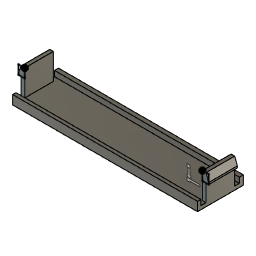
clone-bay-cover-3.5 (Autodesk Fusion 360 design; units mm, degrees)
Autodesk Fusion 360 part; units mm, degrees
sketch "Base" plane through (0, 0, 0) normal (0, 0, 1) x (1, 0, 0)
  line L0 (2, 2) -> (105.25, 2)
  line L1 (105.25, 2) -> (105.25, 27.6)
  line L2 (105.25, 27.6) -> (2, 27.6)
  line L3 (2, 27.6) -> (2, 2)
  dimension "d1" = 25.6
  dimension "d2" = 103.25
  constraint horizontal L0
  constraint vertical L1
  constraint horizontal L2
  constraint vertical L3
  measures "d1" distance of L0.start L2.end
  measures "d2" distance of L0.start L0.end
  measures "d15" distance of L0.start
extrude "Extrude1" add sketch "Base" along normal blind 2
sketch "Rail" plane through (0, 0, 2) normal (0, 0, 1) x (-1, 0, 0)
  line L0 (-2, -27.6) -> (-2, -2)
  line L1 (-2, -2) -> (-105.25, -2)
  line L2 (-105.25, -2) -> (-105.25, -27.6)
  line L3 (-105.25, -27.6) -> (-2, -27.6)
  line L4 (-2, -27.6) -> (-105.25, -27.6)
  line L5 (-105.25, -27.6) -> (-105.25, -25.35)
  line L6 (-105.25, -25.35) -> (-2, -25.35)
  line L7 (-2, -25.35) -> (-2, -27.6)
  line L8 (-2, -2) -> (-105.25, -2)
  line L9 (-105.25, -2) -> (-105.25, -3.88)
  line L10 (-105.25, -3.88) -> (-2, -3.88)
  line L11 (-2, -3.88) -> (-2, -2)
  dimension "d5" = 2.25
  dimension "d6" = 1.88
  constraint horizontal L4
  constraint vertical L5
  constraint horizontal L6
  constraint vertical L7
  constraint coincident L2 L5.end
  constraint coincident L0.start L3.end
  constraint horizontal L8
  constraint vertical L9
  constraint horizontal L10
  constraint vertical L11
  constraint coincident L2 L9.end
  constraint coincident L0.end L1.start
  measures "d5" distance of L4 L6
  measures "d6" distance of L8 L10
extrude "Extrude2" add sketch "Rail" along normal blind 3 contours L0 L2 L3 L4 L5 L6 L7 | L0 L1 L2 L8 L9 L10 L11
sketch "Hook (1.5mm -> 2mm)" plane through (0, 0, 2) normal (0, 0, 1) x (-1, 0, 0)
  line L0 (-2, -3.88) -> (-105.25, -3.88)
  line L1 (-105.25, -3.88) -> (-105.25, -25.35)
  line L2 (-105.25, -25.35) -> (-2, -25.35)
  line L3 (-2, -25.35) -> (-2, -3.88)
  line L4 (-2, -22.75) -> (-4, -22.75)
  line L5 (-4, -22.75) -> (-4, -6.75)
  line L6 (-4, -6.75) -> (-2, -6.75)
  line L7 (-2, -6.75) -> (-2, -22.75)
  line L8 (-105.25, -22.75) -> (-103.25, -22.75)
  line L9 (-103.25, -22.75) -> (-103.25, -6.75)
  line L10 (-103.25, -6.75) -> (-105.25, -6.75)
  line L11 (-105.25, -6.75) -> (-105.25, -22.75)
  dimension "d9" = 2.6
  dimension "d10" = 16
  dimension "d11" = 3.07
  dimension "d12" = 2
  dimension "d13" = 2
  dimension "d14" = 16
  dimension "d15" = 2.6
  dimension "d16" = 2.87
  constraint horizontal L4
  constraint vertical L5
  constraint horizontal L6
  constraint vertical L7
  constraint coincident L3 L4.start
  constraint horizontal L8
  constraint vertical L9
  constraint horizontal L10
  constraint vertical L11
  constraint coincident L1 L8.start
  measures "d9" distance of L2 L4
  measures "d10" distance of L4 L6
  measures "d12" distance of L5 L7
  measures "d13" distance of L8.start L8.end
  measures "d14" distance of L8.start L10.end
  measures "d15" distance of L2 L8.start
  measures "d16" distance of L0 L9.end
extrude "Extrude3" add sketch "Hook (1.5mm -> 2mm)" along normal blind 14.5 contours L3 L4 L5 L6 L7 | L1 L8 L9 L10 L11
sketch "Hook Left" plane through (0, 6.75, 0) normal (0, -1, 0) x (1, 0, 0)
  line L0 (2, 2) -> (4, 2)
  line L1 (4, 2) -> (4, 16.5)
  line L2 (4, 16.5) -> (2, 16.5)
  line L3 (2, 16.5) -> (2, 2)
  line L4 (4, 16.5) -> (0.5, 16.5)
  line L5 (0.5, 16.5) -> (0.5, 11.5)
  line L6 (0.5, 11.5) -> (4, 11.5)
  line L7 (4, 11.5) -> (4, 16.5)
  dimension "d19" = 3.5
  dimension "d20" = 5
  constraint horizontal L4
  constraint vertical L5
  constraint horizontal L6
  constraint vertical L7
  constraint coincident L1.end L2.start
  measures "d19" distance of L1.end L4.end
  measures "d20" distance of L1.end L6.end
sketch "Hook Right" plane through (0, 6.75, 0) normal (0, -1, 0) x (1, 0, 0)
  line L0 (103.25, 2) -> (105.25, 2)
  line L1 (105.25, 2) -> (105.25, 16.5)
  line L2 (105.25, 16.5) -> (103.25, 16.5)
  line L3 (103.25, 16.5) -> (103.25, 2)
  line L4 (103.25, 16.5) -> (106.75, 16.5)
  line L5 (106.75, 16.5) -> (106.75, 11.5)
  line L6 (106.75, 11.5) -> (103.25, 11.5)
  line L7 (103.25, 11.5) -> (103.25, 16.5)
  dimension "d21" = 5
  dimension "d22" = 3.5
  constraint horizontal L4
  constraint vertical L5
  constraint horizontal L6
  constraint vertical L7
  constraint coincident L2.end L3.start
  measures "d21" distance of L2.end L6.end
  measures "d22" distance of L2.end L4.end
extrude "Extrude5" add sketch "Hook Left" sketch "Hook Right" against normal blind 16 contours L3 L4 L5 L6 of sketch 2 contours L1 L4 L5 L6
chamfer "Chamfer1" distance 4 distance2 1.5 1 edges at (0.5, 14.75, 16.5) measured on face at (0.5, 12.0833, 14.8333)
chamfer "Chamfer2" distance 1.5 distance2 4 1 edges at (106.75, 14.75, 16.5) measured on face at (104.4167, 12.0833, 16.5)
extrude "Extrude4" [rolled back] along distance -16 taper angle 0
equation "d19 = 1.5 mm + 2 mm"
equation "d22 = 2 mm + 1.5 mm"
named bodies: "3.5 Cover"
